Wallhanger (Autodesk Fusion 360 design; units mm, degrees)
Autodesk Fusion 360 part; units mm, degrees
sketch "Sketch1" plane through (0, 0, 0) normal (0, 0, 1) x (1, 0, 0)
  line L0 (0, 0) -> (-3, 0)
  line L1 (-3, 0) -> (-3, -8)
  line L2 (-3, -8) -> (0, -8)
  line L3 (0, -8) -> (0, 0)
  line L4 (-5, -8) -> (2, -8)
  line L5 (2, -8) -> (2, 2)
  line L6 (2, 2) -> (-5, 2)
  line L7 (-5, 2) -> (-5, -8)
  line L8 (-2.1, -8) -> (-0.9, -8)
  line L9 (-0.9, -8) -> (-0.9, -1)
  line L10 (-0.9, -1) -> (-2.1, -1)
  line L11 (-2.1, -1) -> (-2.1, -8)
  dimension "d1" = 3
  dimension "d2" = 8
  dimension "d3" = 2
  dimension "d4" = 2
  dimension "d5" = 2
  dimension "d10" = 1.2
  dimension "d12" = 1
  dimension "d13" = 0.9
  constraint horizontal L0
  constraint vertical L1
  constraint horizontal L2
  constraint vertical L3
  constraint coincident L0.start L3.end
  constraint horizontal L4
  constraint vertical L5
  constraint horizontal L6
  constraint vertical L7
  constraint collinear L2 L4
  constraint horizontal L8
  constraint vertical L9
  constraint horizontal L10
  constraint vertical L11
  constraint collinear L4 L8
  measures "d1" distance of L0.start L0.end
  measures "d2" distance of L0.start L2.end
  measures "d3" distance of L1 L7
  measures "d4" distance of L0 L6
  measures "d5" distance of L3 L5
  measures "d10" distance of L8.start L8.end
  measures "d12" distance of L0 L10
  measures "d13" distance of L1 L11
extrude "Extrude1" add sketch "Sketch1" along normal blind 1 contours L0 L1 L2 L3 L4 L9 L10 L11 | L2 L4 L8 L9 L10 L11 makes body 1
extrude "Extrude2" add sketch "Sketch1" along normal blind 2 contours L0 L1 L3 L4 L5 L6 L7 bodies 1
extrude "Extrude3" add sketch "Sketch1" along normal blind 1 from surface at 2 contours L0 L1 L2 L3 L4 L9 L10 L11 | L0 L1 L3 L4 L5 L6 L7 bodies 1
chamfer "Chamfer1" distance 0.9 angle 45 2 edges at (-2.1, -8, 2.5) (-0.9, -8, 2.5) on bodies 1
sketch "Sketch2" plane through (0, 0, 0) normal (0, 0, 1) x (1, 0, 0)
  line L0 (7, 2) -> (22, 2)
  line L1 (22, 2) -> (22, -5)
  line L2 (22, -5) -> (7, -5)
  line L3 (7, -5) -> (7, 2)
  line L4 (7, 2) -> (10, 2)
  line L5 (10, 2) -> (10, -5)
  line L6 (10, -5) -> (7, -5)
  line L7 (7, -5) -> (7, 2)
  line L8 (22, 2) -> (19, 2)
  line L9 (19, 2) -> (19, -5)
  line L10 (19, -5) -> (22, -5)
  line L11 (22, -5) -> (22, 2)
  line L12 (13, 2) -> (16, 2)
  line L13 (16, 2) -> (16, -5)
  line L14 (16, -5) -> (13, -5)
  line L15 (13, -5) -> (13, 2)
  line L16 (7, 2) -> (22, 2)
  line L17 (22, 2) -> (22, 0)
  line L18 (22, 0) -> (7, 0)
  line L19 (7, 0) -> (7, 2)
  dimension "d21" = 15
  dimension "d22" = 2
  constraint horizontal L0
  constraint vertical L1
  constraint horizontal L2
  constraint vertical L3
  constraint horizontal L4
  constraint vertical L5
  constraint horizontal L6
  constraint vertical L7
  constraint coincident L2 L5.end
  constraint horizontal L8
  constraint vertical L9
  constraint horizontal L10
  constraint vertical L11
  constraint coincident L2 L9.end
  constraint horizontal L12
  constraint vertical L13
  constraint horizontal L14
  constraint vertical L15
  constraint coincident L2 L13.end
  constraint coincident L0 L12.start
  constraint horizontal L16
  constraint vertical L17
  constraint horizontal L18
  constraint vertical L19
  measures "d21" distance of L0.start L0.end
  measures "d22" distance of L0.start L18.end
extrude "Extrude5" add sketch "Sketch2" along normal blind 1 separate body makes body 2
extrude "Extrude6" add sketch "Sketch2" along normal blind 3.6 contours L0 L3 L4 L5 L7 L16 L18 L19 | L0 L5 L15 L16 L18 | L0 L12 L13 L15 L16 L18 | L0 L9 L13 L16 L18 | L0 L1 L8 L9 L11 L16 L17 L18 bodies 2
extrude "Extrude7" add sketch "Sketch2" along normal blind 1 from surface at 2.6 contours L2 L3 L5 L6 L7 L18 | L2 L13 L14 L15 L18 | L1 L2 L9 L10 L11 L18 bodies 2
